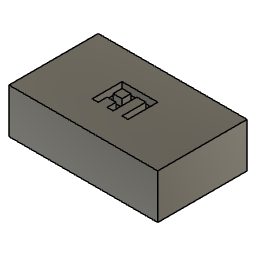
Handschleifklotz v3 (Autodesk Fusion 360 design; units mm, degrees)
Autodesk Fusion 360 part; units mm, degrees
sketch "Skizze1" plane through (0, 0, 0) normal (0, 0, 1) x (1, 0, 0)
  line L0 (50, -30) -> (-50, -30)
  line L1 (-50, -30) -> (-50, 30)
  line L2 (-50, 30) -> (50, 30)
  line L3 (50, 30) -> (50, -30)
  line L4 (50, -30) -> (-50, 30) construction
  line L5 (-50, -30) -> (50, 30) construction
  dimension "d1" = 100
  dimension "d2" = 60
  constraint horizontal L0
  constraint perpendicular L0 L1
  constraint parallel L0 L2
  constraint parallel L1 L3
  constraint coincident L4 origin
  constraint coincident L5 origin
  measures "d1" distance of L1.end L2.end
  measures "d2" distance of L0.end L1.end
extrude "Extrusion1" add sketch "Skizze1" along normal blind 30
sketch "Skizze2" plane through (0, 0, 30) normal (0, 0, 1) x (-1, 0, 0)
  line L0 (-50, -30) -> (50, -30)
  line L1 (50, -30) -> (50, 30)
  line L2 (50, 30) -> (-50, 30)
  line L3 (-50, 30) -> (-50, -30)
  line L4 (10, 10) -> (14, 10)
  line L5 (14, 10) -> (14, -10)
  line L6 (14, -10) -> (10, -10)
  line L7 (0, -6) -> (0, 10)
  line L8 (4, -10) -> (0, -10)
  line L9 (0, 10) -> (4, 10)
  line L10 (-6, 10) -> (-6, -6)
  line L11 (-10, -10) -> (-10, 10)
  line L12 (-6, -10) -> (-10, -10)
  line L13 (-10, 10) -> (-6, 10)
  line L14 (14, -10) -> (-10, -10)
  line L15 (14, -10) -> (14, -6)
  line L16 (10, 0) -> (4, 0)
  line L17 (14, 0) -> (14, 4)
  line L18 (10, 4) -> (4, 4)
  line L19 (10, -6) -> (10, 0)
  line L20 (10, 4) -> (10, 10)
  line L21 (4, 10) -> (4, 4)
  line L22 (4, 0) -> (4, -6)
  line L23 (10, -6) -> (4, -6)
  line L24 (0, -6) -> (-6, -6)
  dimension "d5" = 4
  dimension "d10" = 4
  dimension "d11" = 4
  constraint vertical L19
  constraint perpendicular L4 L19
  constraint perpendicular L4 L5
  constraint perpendicular L5 L6
  constraint perpendicular L14 L15
  constraint perpendicular L11 L23
  constraint midpoint L5 L17.start
  constraint perpendicular L16 L17
  constraint perpendicular L18 L21
  constraint coincident L18.start L19
  constraint collinear L19 L20
  constraint collinear L21 L22
  constraint coincident L16.end L21
  constraint coincident L7.start L23
  constraint collinear L23 L24
  measures "d5" distance of L4.start L4.end
  measures "d10" distance of L5.end L15.end
  measures "d11" distance of L17.start L17.end
extrude "Extrusion2" cut sketch "Skizze2" against normal blind 5 contours L4 L5 L6 L7 L8 L9 L10 L11 L12 L13 L14 L15 L17 L18 L20 L21 L24
